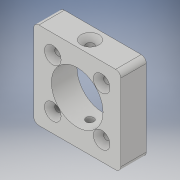
# Autodesk Inventor part: крепление трубы
Saved by Autodesk Inventor 2019.1 (Build 231200000, 200)
## iProperties
Created: 2018-08-22
Part Number: крепление трубы
Material: Типовые
Document SubType Name: Modeling
Designer: Олег
Density: 1 g/cm^3
Appearance: По умолчанию
Author: Олег
Autodesk Inventor part; units mm, degrees
ref_plane "YZ Plane" through (0, 0, 0) normal (1, 0, 0) x (0, 1, 0)
ref_plane "XZ Plane" through (0, 0, 0) normal (0, 1, 0) x (-1, 0, 0)
ref_plane "XY Plane" through (0, 0, 0) normal (0, 0, 1) x (1, 0, 0)
sketch "Эскиз1" plane through (0, 0, 0) normal (0, 0, 1) x (1, 0, 0)
  circle A0 centre (0, 0) radius 13.5 construction
  circle A1 centre (-9.5459, 9.5459) radius 1.25
  line L0 (-9.5459, 9.5459) -> (0, 0) construction
  line L1 (0, 0) -> (2.2284, 0) construction
  circle A2 centre (-9.5459, -9.5459) radius 1.25
  circle A3 centre (9.5459, -9.5459) radius 1.25
  circle A4 centre (9.5459, 9.5459) radius 1.25
  line L2 (17, -17) -> (-17, -17)
  line L3 (-17, -17) -> (-17, 17)
  line L4 (-17, 17) -> (17, 17)
  line L5 (17, 17) -> (17, -17)
  line L6 (17, -17) -> (-17, 17) construction
  line L7 (-17, -17) -> (17, 17) construction
  dimension "d0" = 27
  dimension "d1" = 2.5
  dimension "d3" = 45
  dimension "d6" = 360
  dimension "d8" = 34
  dimension "d9" = 34
  constraints: 16 end point, 4 centre point, 2 coincident, 2 horizontal, 2 midpoint, 2 parallel, 1 perpendicular, 1 point on line, 12 other
  measures "d1" diameter of A1
  measures "d3" angle of L1 L0
  measures "d8" distance of L3.end L4.end
  measures "d9" distance of L2.end L3.end
extrude "Выдавливание1" add sketch "Эскиз1" along normal blind 10
fillet "Сопряжение1" radius 2 4 edges at (17, 17, 5) (-17, 17, 5) (-17, -17, 5) (17, -17, 5)
sketch "Эскиз2" plane through (-15, 17, 0) normal (0, 1, 0) x (1, 0, 0)
  circle A0 centre (15, -5) radius 1.5
  line L0 (-2, 0) -> (-2, -10) projected
  line L1 (0, 0) -> (30, 0) projected
  point P0 (15, 0)
  point P1 (-2, -5)
  point P2 (15, 0)
  dimension "d16" = 3
  constraints: 2 midpoint, 1 centre point, 1 horizontal alignment, 1 vertical alignment
  measures "d16" diameter of A0
sketch "Эскиз3" plane through (0, 0, 10) normal (0, 0, 1) x (1, 0, 0)
  circle A0 centre (0, 0) radius 10.1
  dimension "d13" = 20.2
  constraints: 1 centre point, 1 coincident
  measures "d13" diameter of A0
extrude "Выдавливание2" cut sketch "Эскиз3" against normal blind 10
extrude "Выдавливание3" cut sketch "Эскиз2" against normal blind 40.5
chamfer "Фаска1" distance 2 angle 45 5 edges at (-10.7959, 9.5459, 10) (8.2959, 9.5459, 10) (8.2959, -9.5459, 10) (-10.7959, -9.5459, 10) (-1.5, 17, 5)
